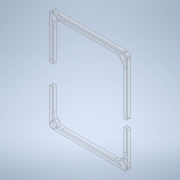
# Autodesk Inventor part: Plex_Rand_untere2
Saved by Autodesk Inventor 2022 (Build 260153000, 153)
## iProperties
Created: 2021-06-16
Part Number: Plex_Rand_untere2
Material: PET Plastic
Document SubType Name: Modeling
Designer: domin
Density: 1.541 g/cm^3
Appearance: Polycarbonate - Clear
Mass: 31.1285 g
Surface Area: 140.669 cm^2
Volume: 20.2002 cm^3
Author: domin
Autodesk Inventor part; units mm, degrees
ref_plane "YZ Plane" through (0, 0, 0) normal (1, 0, 0) x (0, 1, 0)
ref_plane "XZ Plane" through (0, 0, 0) normal (0, 1, 0) x (-1, 0, 0)
ref_plane "XY Plane" through (0, 0, 0) normal (0, 0, 1) x (1, 0, 0)
sketch "Sketch1" plane through (0, 0, 0) normal (0, 0, 1) x (1, 0, 0)
  line L0 (-57, -81) -> (57, -81)
  line L1 (62, -76) -> (62, -22)
  line L2 (57, 81) -> (-57, 81)
  line L3 (-62, 76) -> (-62, 9)
  line L4 (-41, -73) -> (41, -73)
  line L5 (56, -58) -> (56, -22)
  line L6 (41, 73) -> (-41, 73)
  line L7 (-56, 58) -> (-56, 9)
  arc A0 (-56, -58) -> (-41, -73) centre (-41, -58) ccw
  arc A1 (-41, 73) -> (-56, 58) centre (-41, 58) ccw
  arc A2 (56, 58) -> (41, 73) centre (41, 58) ccw
  arc A3 (41, -73) -> (56, -58) centre (41, -58) ccw
  line L8 (56, -22) -> (62, -22)
  line L9 (56, -10) -> (62, -10)
  line L10 (-56, 9) -> (-62, 9)
  line L11 (-62, -22) -> (-56, -22)
  line L12 (-62, -22) -> (-62, -76)
  line L13 (-62, 9) -> (-62, -22) construction
  line L14 (-56, -22) -> (-56, -58)
  line L15 (-56, 9) -> (-56, -22) construction
  line L16 (56, -22) -> (56, -10) construction
  line L17 (56, -10) -> (56, 58)
  line L18 (62, -22) -> (62, -10) construction
  line L19 (62, -10) -> (62, 76)
  arc A4 (-62, -76) -> (-57, -81) centre (-57, -76) ccw
  arc A5 (-57, 81) -> (-62, 76) centre (-57, 76) ccw
  arc A6 (62, 76) -> (57, 81) centre (57, 76) ccw
  arc A7 (57, -81) -> (62, -76) centre (57, -76) ccw
  circle A8 centre (-55, -74) radius 5.25
  line L20 (-92.4325, 0) -> (79.0499, 0) construction
  line L21 (0, -100.3717) -> (0, 120.689) construction
  circle A9 centre (-55, 74) radius 5.25
  circle A10 centre (55, -74) radius 5.25
  circle A11 centre (55, 74) radius 5.25
  point P0 (0, 0)
  point P1 (-62, -81)
  point P2 (62, 81)
  point P3 (-62, 81)
  dimension "d0" = 162
  dimension "d1" = 124
  dimension "d2" = 62
  dimension "d3" = 81
  dimension "d4" = 6
  dimension "d5" = 8
  dimension "d6" = 6
  dimension "d7" = 8
  dimension "d8" = 15
  dimension "d9" = 12
  dimension "d10" = 59
  dimension "d11" = 59
  dimension "d12" = 72
  dimension "d13" = 5
  dimension "d14" = 7
  dimension "d15" = 7
  dimension "d16" = 10.5
  constraints: 44 end point, 24 tangent, 20 parallel, 18 perpendicular, 16 point on circle, 12 centre point, 10 point on line, 6 equal radius, 3 horizontal, 3 symmetric about line, 1 vertical, 3 other
  measures "d0" distance of point (-62, 81) point (-62, -81)
  measures "d1" distance of point (62, 81) point (-62, 81)
  measures "d2" distance from line of L3 point (0, 0)
  measures "d3" distance from line of point (0, 0) L0
  measures "d4" distance between parallel lines of L3 L7
  measures "d5" distance between parallel lines of L0 L4
  measures "d6" distance between parallel lines of L1 L5
  measures "d7" distance between parallel lines of L2 L6
  measures "d8" radius of A0
  measures "d9" distance between parallel lines of L9 L8
  measures "d10" distance between parallel lines of L8 L0
  measures "d11" distance between parallel lines of L0 L11
  measures "d12" distance between parallel lines of L2 L10
  measures "d13" radius of A4
  measures "d14" distance from line of A8.centre L12
  measures "d15" distance from line of A8.centre L0
  measures "d16" diameter of A8
extrude "Extrusion1" add sketch "Sketch1" along normal blind 5
fillet "Fillet1" radius 2 4 edges at (62, -22, 2.5) (62, -10, 2.5) (-62, 9, 2.5) (-62, -22, 2.5)
body "Solid1"
